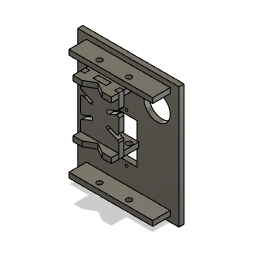
servo (Autodesk Fusion 360 design; units mm, degrees)
Autodesk Fusion 360 part; units mm, degrees
sketch "Sketch1" plane through (0, 0, 0) normal (0, 0, 1) x (1, 0, 0)
  circle A0 centre (0, 0) radius 5.5
  circle A1 centre (34.9, 0) radius 7.49
  line L0 (34.9, 0) -> (0, 0) construction
  dimension "d1" = 34.9
  dimension "d2" = 14.98
  dimension "d3" = 11
  constraint coincident A0.centre L0.end
  constraint coincident A1.centre L0.start
  constraint horizontal L0
  measures "d1" distance of A0.centre A1.centre
  measures "d2" diameter of A1
  measures "d3" diameter of A0
sketch "Sketch2" plane through (0, 0, 0) normal (0, 0, 1) x (1, 0, 0)
  line L0 (23.41, -12.5429) -> (11.41, -12.5429)
  line L1 (11.41, -12.5429) -> (11.41, -35.5429)
  line L2 (11.41, -35.5429) -> (23.41, -35.5429)
  line L3 (23.41, -35.5429) -> (23.41, -12.5429)
  circle A0 centre (34.9, 0) radius 7.49
  line L4 (34.9, 0) -> (0, 0)
  line L5 (23.41, -12.5429) -> (11.41, -35.5429) construction
  line L6 (23.41, -35.5429) -> (11.41, -12.5429) construction
  line L7 (17.41, 17.6056) -> (17.41, -18.0173) construction
  circle A1 centre (17.41, -10.2429) radius 1 construction
  circle A2 centre (17.41, -10.2429) radius 0.75
  circle A3 centre (17.41, -37.8429) radius 0.75
  circle A4 centre (17.41, -37.8429) radius 1 construction
  line L8 (-10.5, 16.19) -> (47.39, 16.19)
  line L9 (47.39, 16.19) -> (47.39, -53.3429)
  line L10 (47.39, -53.3429) -> (-10.5, -53.3429)
  line L11 (-10.5, -53.3429) -> (-10.5, 16.19)
  circle A5 centre (0, 0) radius 5.5
  circle A6 centre (17.41, -18.5429) radius 6 construction
  circle A7 centre (17.41, -29.5429) radius 6 construction
  circle A8 centre (17.41, -29.5429) radius 18 construction
  circle A9 centre (17.41, -18.5429) radius 18 construction
  line L12 (23.41, -24.0429) -> (11.41, -24.0429) construction
  point P0 (17.41, -24.0429)
  dimension "d5" = 23
  dimension "d6" = 12
  dimension "d7" = 4
  dimension "d9" = 2
  dimension "d10" = 1.5
  dimension "d11" = 25.6
  dimension "d12" = 5
  dimension "d13" = 5
  dimension "d61" = 11.91
  dimension "d62" = 36
  dimension "d63" = 14.5
  dimension "d64" = 8.7
  constraint horizontal L0
  constraint vertical L1
  constraint horizontal L2
  constraint vertical L3
  constraint midpoint L5 P0
  constraint coincident P0 L7
  constraint vertical L7
  constraint coincident L7 A1.centre
  constraint concentric A1 A2
  constraint horizontal L8
  constraint vertical L9
  constraint horizontal L10
  constraint vertical L11
  constraint tangent L3 A6
  constraint tangent L0 A6
  constraint tangent L1 A6
  constraint tangent L3 A7
  constraint tangent L2 A7
  constraint tangent L1 A7
  constraint concentric A7 A8
  constraint concentric A6 A9
  constraint equal A8 A9
  constraint midpoint L3 L12.start
  constraint midpoint L1 L12.end
  constraint symmetric A2 A3 L12
  constraint symmetric A1 A4 L12
  constraint tangent A0 A9
  measures "d5" distance of L0.start L2.end
  measures "d6" distance of L0.start L0.end
  measures "d7" distance of L3 A0
  measures "d9" diameter of A1
  measures "d10" diameter of A2
  measures "d11" distance of A1 A4
  measures "d12" distance of A0 L9
  measures "d13" distance of L11 A5
  measures "d61" distance of L7 A5
  measures "d62" diameter of A8
  measures "d63" distance of A4 L10
  measures "d64" distance of A0 L8
extrude "Extrude1" add sketch "Sketch2" along normal blind 2.9 makes body 1
sketch "Sketch3" plane through (0, 16.19, 0) normal (0, 1, 0) x (-1, 0, 0)
  line L0 (-47.39, 0) -> (10.5, 0)
  line L1 (10.5, 0) -> (10.5, 2.9)
  line L2 (10.5, 2.9) -> (-47.39, 2.9)
  line L3 (-47.39, 2.9) -> (-47.39, 0)
  line L4 (-42.39, 2.9) -> (-27.41, 2.9)
  line L5 (-5.5, 2.9) -> (5.5, 2.9)
  line L6 (-11.41, 2.9) -> (-23.41, 2.9)
  line L7 (-42.39, 2.9) -> (5.5, 2.9)
  line L8 (5.5, 2.9) -> (5.5, 12.9)
  line L9 (5.5, 12.9) -> (-42.39, 12.9)
  line L10 (-42.39, 12.9) -> (-42.39, 2.9)
  line L11 (-23.41, 2.9) -> (-27.41, 2.9) construction
  line L12 (-25.41, 2.9) -> (-25.41, 12.9) construction
  line L13 (-5.5, 2.9) -> (-11.41, 2.9) construction
  line L14 (-8.455, 2.9) -> (-8.455, 12.9) construction
  circle A0 centre (-25.41, 9.4) radius 1.5
  circle A1 centre (-8.455, 9.4) radius 1.5
  line L15 (-42.39, 2.9) -> (5.5, 2.9)
  line L16 (5.5, 2.9) -> (5.5, 0)
  line L17 (5.5, 0) -> (-42.39, 0)
  line L18 (-42.39, 0) -> (-42.39, 2.9)
  line L19 (10.5, 0) -> (-47.39, 0)
  line L20 (-30.3959, 5.9) -> (-5.6168, 5.9) construction
  dimension "d18" = 10
  dimension "d19" = 3
  dimension "d26" = 2
  dimension "d27" = 2
  dimension "d29" = 2
  constraint horizontal L7
  constraint vertical L8
  constraint horizontal L9
  constraint vertical L10
  constraint coincident L4.start L7.start
  constraint coincident L5.end L8
  constraint coincident L6.end L11.start
  constraint coincident L4.end L11.end
  constraint midpoint L11 L12.start
  constraint coincident L9 L12.end
  constraint perpendicular L9 L12
  constraint coincident L5.start L13.start
  constraint coincident L6.start L13.end
  constraint midpoint L13 L14.start
  constraint coincident L9 L14.end
  constraint perpendicular L9 L14
  constraint equal A0 A1
  constraint horizontal L15
  constraint vertical L16
  constraint horizontal L17
  constraint vertical L18
  constraint coincident L0 L16.end
  constraint collinear L8 L16
  constraint coincident L12 A0.centre
  constraint coincident L14 A1.centre
  constraint horizontal L20
  measures "d18" distance of L4.start L9.end
  measures "d19" diameter of A0
  measures "d26" distance of L9 A0
  measures "d27" distance of L9 A1
  measures "d29" distance of A0 L20
extrude "Extrude2" add sketch "Sketch3" against normal blind 2.9 from surface at -2.9 separate body contours L0 L2 L4 L5 L6 L7 L15 L16 L17 L18 L19 | L2 L4 L5 L6 L7 L8 L9 L10 L15 makes body 2
sketch "Sketch4" plane through (0, 0, 0) normal (0, 0, -1) x (-1, 0, 0)
  line L0 (5.5, 13.29) -> (-42.39, 13.29)
  line L1 (-42.39, 13.29) -> (-42.39, 10.39)
  line L2 (-42.39, 10.39) -> (5.5, 10.39)
  line L3 (5.5, 10.39) -> (5.5, 13.29)
  line L4 (-20.945, 13.29) -> (-15.945, 13.29)
  line L5 (-15.945, 13.29) -> (-15.945, 10.39)
  line L6 (-15.945, 10.39) -> (-20.945, 10.39)
  line L7 (-20.945, 10.39) -> (-20.945, 13.29)
  line L8 (-18.445, 13.29) -> (-18.445, 10.39) construction
  dimension "d23" = 5
  constraint horizontal L4
  constraint vertical L5
  constraint horizontal L6
  constraint vertical L7
  constraint coincident L2 L5.end
  constraint coincident L0 L4.start
  constraint midpoint L0 L8.start
  constraint midpoint L2 L8.end
  constraint symmetric L5 L7 L8
  measures "d23" distance of L4.start L4.end
extrude "Extrude3" cut sketch "Sketch4" against normal blind 2.9 contours L0 L2 L4 L5 L6 L7 bodies 2
pattern_linear "R-Pattern1" count 3 spacing 15 along (-1, 0, 0) both ways of "Extrude3"
ref_plane "WorkPlane2" through (18.445, -18.5765, 1.45) normal (0, 1, 0) x (-1, 0, 0)
mirror "Mirror1" about plane through (18.445, -18.5765, 1.45) normal (0, 1, 0) of bodies 2 makes body 3
combine "Combine1" operation cut target body 1 tool bodies 3 2 keep tools
sketch "Sketch5" plane through (0, 10.39, 0) normal (0, -1, 0) x (1, 0, 0)
  line L0 (5.945, 2.9) -> (5.945, 0)
  line L1 (5.945, 0) -> (15.945, 0)
  line L2 (15.945, 0) -> (15.945, 2.9)
  line L3 (15.945, 2.9) -> (20.945, 2.9)
  line L4 (20.945, 2.9) -> (20.945, 0)
  line L5 (20.945, 0) -> (30.945, 0)
  line L6 (30.945, 0) -> (30.945, 2.9)
  line L7 (30.945, 2.9) -> (35.945, 2.9)
  line L8 (35.945, 2.9) -> (35.945, 0)
  line L9 (35.945, 0) -> (42.39, 0)
  line L10 (42.39, 0) -> (42.39, 12.9)
  line L11 (42.39, 12.9) -> (-5.5, 12.9)
  line L12 (-5.5, 12.9) -> (-5.5, 0)
  line L13 (-5.5, 0) -> (0.945, 0)
  line L14 (0.945, 0) -> (0.945, 2.9)
  line L15 (0.945, 2.9) -> (5.945, 2.9)
  circle A0 centre (25.41, 9.4) radius 1.5
  circle A1 centre (8.455, 9.4) radius 1.5
  line L16 (5.5, 21.6) -> (27.41, 21.6)
  line L17 (27.41, 21.6) -> (27.41, 5.9)
  line L18 (27.41, 5.9) -> (5.5, 5.9)
  line L19 (5.5, 5.9) -> (5.5, 21.6)
  circle A2 centre (25.41, 9.4) radius 1.575
  circle A3 centre (8.455, 9.4) radius 1.575
  line L20 (-5.5, 2.9) -> (5.5, 2.9)
  line L21 (27.41, 2.9) -> (42.39, 2.9)
  line L22 (5.5, 2.9) -> (5.5, 7) construction
  line L23 (27.41, 2.9) -> (27.41, 8) construction
  line L24 (5.5, 18.3) -> (27.41, 18.3) construction
  line L25 (16.455, 18.3) -> (16.455, 21.6) construction
  line L26 (16.455, 18.3) -> (10.7392, 21.6)
  line L27 (16.455, 18.3) -> (22.1708, 21.6)
  line L28 (27.41, 17.3) -> (5.5, 17.3) construction
  line L29 (16.455, 18.3) -> (16.455, 17.3)
  point P0 (16.455, 17.3)
  dimension "d36" = 2
  dimension "d39" = 8.7
  dimension "d55" = 3.15
  dimension "d66" = 5.4
  dimension "d67" = 60
  dimension "d85" = 1
  constraint horizontal L16
  constraint vertical L17
  constraint horizontal L18
  constraint vertical L19
  constraint concentric A0 A2
  constraint concentric A1 A3
  constraint coincident L20.end L22.start
  constraint perpendicular L18 L22
  constraint coincident L21.start L23.start
  constraint perpendicular L21 L23
  constraint collinear L17 L23
  constraint collinear L19 L22
  constraint coincident L19 L24.start
  constraint coincident L17 L24.end
  constraint perpendicular L17 L24
  constraint midpoint L24 L25.start
  constraint midpoint L16 L25.end
  constraint coincident L16 L26.end
  constraint symmetric L26.start L25 L27.start
  constraint symmetric L25 L26.end L27.end
  constraint equal A2 A3
  constraint coincident L17 L28.start
  constraint coincident L19 L28.end
  constraint perpendicular L19 L28
  constraint midpoint L28 P0
  constraint coincident P0 L29.end
  measures "d36" distance of A1 L18
  measures "d39" distance of L11 L16
  measures "d55" diameter of A2
  measures "d66" distance of L11 L24
  measures "d67" angle of L25 L26
  measures "d85" distance of L24 L28
ref_plane "WorkPlane1" through (25.41, -19.61, 9.4) normal (0, -1, 0) x (1, 0, 0)
extrude "Extrude4" add sketch "Sketch5" along normal blind 2.9 separate body contours L11 L16 L17 L19 L26 L27 | L11 L17 L18 L19 makes body 4
extrude "Extrude5" add sketch "Sketch5" along normal blind 2.9 from surface at 30 separate body contours L11 L16 L17 L19 L26 L27 | L11 L17 L18 L19 makes body 5
ref_plane "WorkPlane3" through (8.1196, 8.94, 17.3) normal (0, 0, 1) x (-1, 0, 0)
sketch "Sketch6" plane through (0, 0, 17.3) normal (0, 0, 1) x (1, 0, 0)
  line L0 (10.655, 10.39) -> (5.5, 10.39)
  line L1 (5.5, 10.39) -> (5.5, 7.49)
  line L2 (5.5, 7.49) -> (10.655, 7.49)
  line L3 (27.41, 7.49) -> (27.41, 10.39)
  line L4 (27.41, -22.51) -> (5.5, -22.51)
  line L5 (5.5, 10.39) -> (27.41, 10.39)
  line L6 (27.41, 10.39) -> (27.41, -22.51)
  line L7 (27.41, -22.51) -> (5.5, -22.51)
  line L8 (5.5, -22.51) -> (5.5, 10.39)
  line L9 (27.41, -6.06) -> (5.5, -6.06) construction
  line L10 (16.455, 10.39) -> (16.455, -22.51) construction
  line L11 (7.8054, 10.39) -> (12.8054, 10.39)
  line L12 (12.8054, 10.39) -> (12.8054, 7.49)
  line L13 (12.8054, 7.49) -> (7.8054, 7.49)
  line L14 (7.8054, 7.49) -> (7.8054, 10.39)
  line L15 (25.1046, 10.39) -> (20.1046, 10.39)
  line L16 (20.1046, 10.39) -> (20.1046, 7.49)
  line L17 (25.1046, 7.49) -> (25.1046, 10.39)
  line L18 (20.1046, 7.49) -> (25.1046, 7.49)
  line L19 (7.8054, -22.51) -> (12.8054, -22.51)
  line L20 (12.8054, -22.51) -> (12.8054, -19.61)
  line L21 (12.8054, -19.61) -> (7.8054, -19.61)
  line L22 (7.8054, -19.61) -> (7.8054, -22.51)
  line L23 (25.1046, -22.51) -> (20.1046, -22.51)
  line L24 (20.1046, -22.51) -> (20.1046, -19.61)
  line L25 (25.1046, -19.61) -> (25.1046, -22.51)
  line L26 (20.1046, -19.61) -> (25.1046, -19.61)
  line L27 (5.5, -8.56) -> (5.5, -3.56)
  circle A0 centre (5.5, -6.06) radius 5
  line L28 (27.41, -8.56) -> (27.41, -3.56)
  circle A1 centre (27.41, -6.06) radius 5
  line L29 (7.4377, -1.4507) -> (12.455, -3.56)
  line L30 (7.4377, -10.6693) -> (12.455, -8.56)
  line L31 (5.5, 1.5334) -> (12.455, -1.3905)
  line L32 (12.455, -1.3905) -> (12.455, -3.56)
  line L33 (5.5, -13.6534) -> (12.455, -10.7295)
  line L34 (12.455, -10.7295) -> (12.455, -8.56)
  line L35 (27.41, 1.5334) -> (20.455, -1.3905)
  line L36 (20.455, -1.3905) -> (20.455, -3.56)
  line L37 (25.4723, -1.4507) -> (20.455, -3.56)
  line L38 (25.4723, -10.6693) -> (20.455, -8.56)
  line L39 (27.41, -13.6534) -> (20.455, -10.7295)
  line L40 (20.455, -10.7295) -> (20.455, -8.56)
  line L41 (10.655, 7.49) -> (10.655, 10.39)
  line L42 (27.41, 10.39) -> (22.255, 10.39)
  line L43 (22.255, 10.39) -> (22.255, 7.49)
  line L44 (22.255, 7.49) -> (27.41, 7.49)
  dimension "d46" = 2.9
  dimension "d47" = 5
  dimension "d49" = 10
  dimension "d58" = 5
  dimension "d59" = 4
  dimension "d60" = 2
  constraint horizontal L5
  constraint vertical L6
  constraint horizontal L7
  constraint vertical L8
  constraint coincident L4.start L6.end
  constraint coincident L0.end L1.start
  constraint midpoint L6 L9.start
  constraint midpoint L8 L9.end
  constraint midpoint L5 L10.start
  constraint midpoint L4 L10.end
  constraint horizontal L11
  constraint vertical L12
  constraint horizontal L13
  constraint vertical L14
  constraint coincident L5 L11.start
  constraint symmetric L10 L11.start L15.start
  constraint symmetric L10 L11.end L15.end
  constraint symmetric L10 L12.end L16.end
  constraint symmetric L10 L13.end L17.start
  constraint symmetric L9 L11.start L19.start
  constraint symmetric L9 L11.end L19.end
  constraint symmetric L9 L12.end L20.end
  constraint symmetric L9 L13.end L21.end
  constraint symmetric L9 L15.start L23.start
  constraint symmetric L9 L15.end L23.end
  constraint symmetric L9 L16.end L24.end
  constraint symmetric L9 L17.start L25.start
  constraint vertical L27
  constraint midpoint L27 L9.end
  constraint collinear L8 L27
  constraint symmetric L10 L27.end L28.end
  constraint symmetric L10 L27.start L28.start
  constraint symmetric L10 A0 A1
  constraint coincident A0 L29.start
  constraint tangent A0 L29
  constraint coincident L9 A0.centre
  constraint coincident A0 L30.start
  constraint equal L29 L30
  constraint tangent A0 L30
  constraint symmetric L9 L29.end L30.end
  constraint parallel L29 L31
  constraint vertical L32
  constraint coincident L8 L31.start
  constraint symmetric L9 L31.start L33.start
  constraint symmetric L9 L31.end L33.end
  constraint symmetric L10 L29.start L37.start
  constraint symmetric L10 L29.end L36.end
  constraint symmetric L10 L30.start L38.start
  constraint symmetric L10 L30.end L38.end
  constraint symmetric L10 L31.start L35.start
  constraint symmetric L10 L31.end L35.end
  constraint symmetric L10 L33.start L39.start
  constraint symmetric L10 L33.end L39.end
  measures "d46" distance of L11.start L13.end
  measures "d47" distance of L12 L14
  measures "d49" diameter of A0
  measures "d58" vertical distance of L29.end L30.end
  measures "d59" distance of L10 L29.end
  measures "d60" distance of L29 L31
extrude "Extrude6" add sketch "Sketch6" against normal blind 2.9 separate body contours L0 L1 L2 L5 L8 L14 | L2 L4 L5 L6 L7 L8 L12 L13 L16 L18 L20 L21 L22 L24 L25 L26 A0 A1 L29 L30 L31 L32 L33 L34 L35 L36 L37 L38 L39 L40 L44 | L3 L5 L6 L17 L42 L44 | L8 L27 A0 | L6 L28 A1 picked at (7.1667, -6.06) picked at (25.7433, -6.06) makes body 6
combine "Combine2" operation cut target body 4 tool bodies 6 keep tools
combine "Combine3" operation cut target body 5 tool bodies 6 keep tools
fillet "Fillet1" radius 1 16 edges at (27.41, -1.06, 15.85) (27.41, -11.06, 15.85) (20.455, -8.56, 15.85) (20.455, -10.7295, 15.85) (27.41, -13.6534, 15.85) (20.455, -3.56, 15.85) (20.455, -1.3905, 15.85) (27.41, 1.5334, 15.85) (12.455, -3.56, 15.85) (12.455, -1.3905, 15.85) (5.5, -1.06, 15.85) (5.5, -11.06, 15.85) (5.5, -13.6534, 15.85) (5.5, 1.5334, 15.85) (12.455, -8.56, 15.85) (12.455, -10.7295, 15.85) on bodies 6
sketch "Sketch7" plane through (0, 0, 0) normal (0, 0, -1) x (-1, 0, 0)
  line L0 (-0.945, 10.39) -> (-0.945, 13.29)
  line L1 (-0.945, 13.29) -> (5.5, 13.29)
  line L2 (5.5, 13.29) -> (5.5, 10.39)
  line L3 (5.5, 10.39) -> (-0.945, 10.39)
  line L4 (-5.945, 13.29) -> (-5.945, 10.39)
  line L5 (-5.945, 10.39) -> (-15.945, 10.39)
  line L6 (-15.945, 10.39) -> (-15.945, 13.29)
  line L7 (-15.945, 13.29) -> (-5.945, 13.29)
  line L8 (-42.39, 13.29) -> (-35.945, 13.29)
  line L9 (-35.945, 13.29) -> (-35.945, 10.39)
  line L10 (-35.945, 10.39) -> (-42.39, 10.39)
  line L11 (-42.39, 10.39) -> (-42.39, 13.29)
  line L12 (-30.945, 13.29) -> (-20.945, 13.29)
  line L13 (-20.945, 13.29) -> (-20.945, 10.39)
  line L14 (-20.945, 10.39) -> (-30.945, 10.39)
  line L15 (-30.945, 10.39) -> (-30.945, 13.29)
  line L16 (-0.945, -50.4429) -> (-0.945, -47.5429)
  line L17 (-0.945, -47.5429) -> (5.5, -47.5429)
  line L18 (5.5, -47.5429) -> (5.5, -50.4429)
  line L19 (5.5, -50.4429) -> (-0.945, -50.4429)
  line L20 (-5.945, -47.5429) -> (-5.945, -50.4429)
  line L21 (-5.945, -50.4429) -> (-15.945, -50.4429)
  line L22 (-15.945, -50.4429) -> (-15.945, -47.5429)
  line L23 (-15.945, -47.5429) -> (-5.945, -47.5429)
  line L24 (-20.945, -50.4429) -> (-30.945, -50.4429)
  line L25 (-30.945, -50.4429) -> (-30.945, -47.5429)
  line L26 (-30.945, -47.5429) -> (-20.945, -47.5429)
  line L27 (-20.945, -47.5429) -> (-20.945, -50.4429)
  line L28 (-35.945, -50.4429) -> (-42.39, -50.4429)
  line L29 (-42.39, -50.4429) -> (-42.39, -47.5429)
  line L30 (-42.39, -47.5429) -> (-35.945, -47.5429)
  line L31 (-35.945, -47.5429) -> (-35.945, -50.4429)
  circle A0 centre (-17.41, -37.8429) radius 0.75
  line L32 (-23.41, -35.5429) -> (-23.41, -12.5429)
  line L33 (-23.41, -12.5429) -> (-11.41, -12.5429)
  line L34 (-11.41, -12.5429) -> (-11.41, -35.5429)
  line L35 (-11.41, -35.5429) -> (-23.41, -35.5429)
  circle A1 centre (-17.41, -10.2429) radius 0.75
  circle A2 centre (-34.9, 0) radius 7.49
  circle A3 centre (0, 0) radius 5.5
  line L36 (-47.39, -53.3429) -> (10.5, -53.3429)
  line L37 (10.5, -53.3429) -> (10.5, 16.19)
  line L38 (10.5, 16.19) -> (-47.39, 16.19)
  line L39 (-47.39, 16.19) -> (-47.39, -53.3429)
ref_plane "WorkPlane4" through (18.445, -18.5765, -12.5) normal (0, 0, -1) x (-1, 0, 0)
sketch "Sketch8" plane through (18.445, -14.2265, -12.5) normal (0, 0, -1) x (1, 0, 0)
  circle A0 centre (-18.445, -14.2265) radius 5.5
  circle A1 centre (-12.6715, -24.2265) radius 2.25 construction
  circle A2 centre (-12.6715, -4.2265) radius 2.25 construction
  circle A3 centre (-29.992, -14.2265) radius 2.25 construction
  line L0 (-12.6715, -24.2265) -> (-12.6715, -4.2265) construction
  line L1 (-14.392, -5.6765) -> (-10.951, -5.6765)
  line L2 (-14.392, -2.7765) -> (-10.951, -2.7765)
  line L3 (-14.392, -5.6765) -> (-14.392, -2.7765)
  line L4 (-10.951, -5.6765) -> (-10.951, -2.7765)
  line L5 (-16.695, -14.2265) -> (4.055, -14.2265)
  line L6 (-14.392, -25.6765) -> (-10.951, -25.6765)
  line L7 (-14.392, -22.7765) -> (-14.392, -25.6765)
  line L8 (-14.392, -22.7765) -> (-10.951, -22.7765)
  line L9 (-10.951, -22.7765) -> (-10.951, -25.6765)
  dimension "d72" = 4.5
  dimension "d74" = 360
  dimension "d75" = 15.5
  dimension "d76" = 2.9
  constraint coincident A1.centre L0.start
  constraint coincident A2.centre L0.end
  constraint vertical L0
  constraint coincident A2 L1.start
  constraint coincident A2 L1.end
  constraint horizontal L1
  constraint coincident A2 L2.start
  constraint coincident A2 L2.end
  constraint horizontal L2
  constraint equal L1 L2
  constraint symmetric L1.start L5 L7.start
  constraint symmetric L1.end L5 L8.end
  constraint symmetric L2.start L5 L6.start
  constraint symmetric L2.end L5 L6.end
  measures "d72" diameter of A1
  measures "d75" distance of A1 A2
  measures "d76" distance of L1 L2
ref_plane "WorkPlane5" through (18.445, -8.55, 1.45) normal (0, -1, 0) x (1, 0, 0)
sketch "Sketch9" plane through (18.445, -8.55, 1.45) normal (0, -1, 0) x (1, 0, 0)
  line L0 (-28.945, 1.45) -> (28.945, 1.45)
  line L1 (28.945, -1.45) -> (-28.945, -1.45)
  line L2 (-10.951, -13.95) -> (-10.951, 1.45)
  line L3 (-26.8807, -1.45) -> (-26.8807, 1.45)
  line L4 (-14.392, -13.95) -> (-14.392, -16.85)
  line L5 (-14.392, -16.85) -> (-10.951, -16.85)
  line L6 (-10.951, -16.85) -> (-10.951, -13.95)
  line L7 (-16.0636, 1.45) -> (-16.0636, -1.45)
  line L8 (-20.8264, -1.45) -> (-20.8264, 1.45)
  line L9 (-18.445, 0.3) -> (-18.445, 21.05)
  line L10 (-14.392, -13.95) -> (-16.392, -13.95)
  line L11 (-16.392, -13.95) -> (-26.8807, -1.45)
  point P0 (-10.951, -13.95)
  point P1 (-14.392, -13.95)
  dimension "d79" = 2.9
  dimension "d82" = 2
  dimension "d83" = 50
  constraint coincident P0 L2.start
  constraint coincident L0 L2.end
  constraint perpendicular L0 L2
  constraint coincident L1 L3.start
  constraint coincident L0 L3.end
  constraint perpendicular L0 L3
  constraint coincident P1 L4.start
  constraint vertical L4
  constraint perpendicular L4 L5
  constraint perpendicular L5 L6
  constraint coincident L0 L7.start
  constraint coincident L1 L7.end
  constraint perpendicular L1 L7
  constraint coincident L1 L8.start
  constraint coincident L0 L8.end
  constraint perpendicular L0 L8
  constraint symmetric L7 L8 L9
  constraint perpendicular L4 L10
  measures "d79" distance of P1 L4.end
  measures "d82" distance of P1 L10.end
  measures "d83" angle of L1 L11
extrude "Extrude7" add sketch "Sketch9" along normal blind 2.9 separate body contours L0 L1 L3 L8 | L1 L2 L4 L5 L6 L10 L11 | L0 L1 L2 L7 makes body 7
ref_plane "WorkPlane6" through (-0.4709, 0, -6.25) normal (0, -1, 0) x (0, 0, -1)
combine "Combine4" operation cut target body 1 tool bodies 7 keep tools
equation "mdfT = 2.9 mm"
equation "d13 = d12"
equation "d14 = 12 mm + 2 * mdfT"
equation "d16 = mdfT"
equation "d20 = -mdfT"
equation "d21 = -mdfT"
equation "d24 = -mdfT"
equation "d27 = d26"
equation "d29 = d26"
equation "d39 = 3 * mdfT"
equation "d41 = mdfT"
equation "d44 = mdfT"
equation "d46 = mdfT"
equation "d53 = -mdfT"
equation "d62 = ( 2 * 18 ) * 1 mm"
equation "d63 = 5 * mdfT"
equation "d64 = 3 * mdfT"
equation "d66 = mdfT + 2.5 mm"
equation "d76 = mdfT"
equation "d79 = mdfT"
equation "d80 = mdfT"
